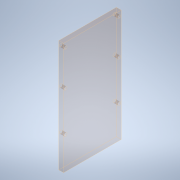
# Autodesk Inventor part: Small_Side_Piece_Final
Saved by Autodesk Inventor 2022 (Build 260153000, 153)
## iProperties
Created: 2023-01-11
Part Number: Small_Side_Piece_Final
Material: Polycarbonate, Smoke
Document SubType Name: Modeling
Designer: s151859
Density: 1.2 g/cm^3
Appearance: Polycarbonate - Smoked
Mass: 122.903 g
Surface Area: 314.387 cm^2
Volume: 102.419 cm^3
Author: s151859
Autodesk Inventor part; units mm, degrees
ref_plane "YZ Plane" through (0, 0, 0) normal (1, 0, 0) x (0, 1, 0)
ref_plane "XZ Plane" through (0, 0, 0) normal (0, 1, 0) x (-1, 0, 0)
ref_plane "XY Plane" through (0, 0, 0) normal (0, 0, 1) x (1, 0, 0)
sketch "Sketch1" plane through (0, 0, 0) normal (0, 1, 0) x (-1, 0, 0)
  line L0 (7.9123, 37.1675) -> (0.2923, 37.1675)
  line L1 (0.2923, 37.1675) -> (0.2923, -54.2725)
  line L2 (0.2923, -54.2725) -> (7.9123, -54.2725)
  line L3 (7.9123, -54.2725) -> (7.9123, 37.1675)
  point P0 (0, 0)
  dimension "d12" = 91.44
  dimension "d13" = 7.62
  constraints: 8 end point, 2 parallel, 1 horizontal, 1 perpendicular
  measures "d12" distance of L0.end L1.end
  measures "d13" distance of L0.start L0.end
extrude "Extrusion1" add sketch "Sketch1" along normal blind 177.8
sketch "Sketch3" plane through (-0.2923, 0, 37.1675) normal (1, 0, 0) x (0, 0, -1)
  circle A0 centre (3.175, 170.18) radius 2.3859
  line L0 (0, 0) -> (0, 177.8) projected
  line L1 (0, 177.8) -> (91.44, 177.8) projected
  circle A1 centre (88.265, 170.18) radius 2.3846
  line L2 (91.44, 0) -> (91.44, 177.8) projected
  circle A2 centre (3.175, 114.3) radius 2.3895
  circle A3 centre (88.265, 114.3) radius 2.3896
  circle A4 centre (3.175, 50.8) radius 2.3895
  circle A5 centre (88.265, 50.8) radius 2.3895
  point P0 (37.1675, 0)
  dimension "d2" = 3.175
  dimension "d3" = 7.62
  dimension "d4" = 7.62
  dimension "d5" = 3.175
  dimension "d6" = 3.175
  dimension "d7" = 3.175
  dimension "d8" = 63.5
  dimension "d9" = 63.5
  dimension "d14" = 3.175
  dimension "d15" = 3.175
  dimension "d16" = 127
  dimension "d17" = 127
  constraints: 6 centre point
  measures "d2" distance from line of L0 A0.centre
  measures "d3" distance from line of L1 A0.centre
  measures "d4" distance from line of L1 A1.centre
  measures "d5" distance from line of A1.centre L2
  measures "d6" distance from line of L0 A2.centre
  measures "d7" distance from line of L2 A3.centre
  measures "d8" distance from line of L1 A3.centre
  measures "d9" distance from line of A2.centre L1
  measures "d14" distance from line of L0 A4.centre
  measures "d15" distance from line of L2 A5.centre
  measures "d16" distance from line of L1 A4.centre
  measures "d17" distance from line of L1 A5.centre
extrude "Extrusion2" cut sketch "Sketch3" against normal blind 11.1125
body "Solid1"
